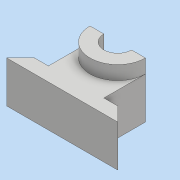
# Autodesk Inventor part: 1
Saved by Autodesk Inventor 2017 (Build 210142000, 142)
## iProperties
Part Number: 1
Material: 一般
Document SubType Name: Modeling
Designer: d8910
Density: 1 g/cm^3
Appearance: 預設
Author: d8910
Autodesk Inventor part; units mm, degrees
ref_plane "YZ Plane" through (0, 0, 0) normal (1, 0, 0) x (0, 1, 0)
ref_plane "XZ Plane" through (0, 0, 0) normal (0, 1, 0) x (-1, 0, 0)
ref_plane "XY Plane" through (0, 0, 0) normal (0, 0, 1) x (1, 0, 0)
sketch "草圖1" plane through (0, 0, 0) normal (0, 0, 1) x (1, 0, 0)
  line L0 (-20, -5) -> (0, -5)
  line L1 (-20, -5) -> (-15, 0)
  line L2 (-15, 0) -> (-10, 0)
  line L3 (-10, 0) -> (-10, 15)
  line L4 (-10, 15) -> (0, 15)
  line L5 (0, -5) -> (0, 15)
  point P0 (0, 0)
  dimension "d0" = 20
  dimension "d1" = 5
  dimension "d2" = 5
  dimension "d3" = 20
  dimension "d4" = 10
  constraints: 12 end point, 2 horizontal, 2 perpendicular, 1 horizontal alignment, 1 vertical, 1 vertical alignment
  measures "d0" distance of L0.start L0.end
  measures "d1" distance between parallel lines of L2 L0
  measures "d2" horizontal distance of L0.start L1.end
  measures "d3" distance between parallel lines of L0 L4
  measures "d4" distance of L3.end L4.end
extrude "擠出1" add sketch "草圖1" along normal mid plane 15
mirror "鏡射1" about plane through (0, -5, 0) normal (1, 0, 0) of "擠出1"
sketch "草圖2" plane through (0, 0, 7.5) normal (0, 0, 1) x (1, 0, 0)
  line L0 (-20, -5) -> (20, -5) construction
  line L1 (15, 0) -> (20, -5) construction
  line L2 (10, 0) -> (15, 0) construction
  line L3 (10, 15) -> (10, 0) construction
  line L4 (-10, 15) -> (10, 15) construction
  line L5 (-10, 15) -> (-10, 0) construction
  line L6 (-10, 0) -> (-15, 0) construction
  line L7 (-15, 0) -> (-20, -5) construction
  line L8 (-10, 15) -> (10, 15) projected
  arc A0 (-10, 15) -> (10, 15) centre (0, 15) ccw
  arc A1 (-5, 15) -> (5, 15) centre (0, 15) ccw
  point P0 (0, 0)
  dimension "d7" = 10
  constraints: 4 point on circle, 2 centre point, 2 end point, 2 point on line, 1 coincident, 1 midpoint
  measures "d7" diameter of A1
extrude "擠出2" add sketch "草圖2" along normal blind 5 contours L8 A1 A0
sketch "草圖3" plane through (0, 0, 7.5) normal (0, 0, 1) x (1, 0, 0)
  arc A0 (-5, 15) -> (5, 15) centre (0, 15) ccw projected
  line L0 (-5, 15) -> (5, 15) projected
  point P0 (0, 0)
extrude "擠出3" cut sketch "草圖3" against normal through all
